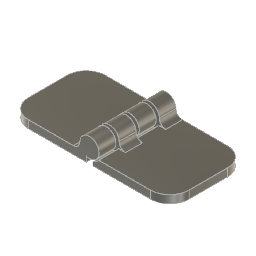
hinge (Autodesk Fusion 360 design; units mm, degrees)
Autodesk Fusion 360 part; units mm, degrees
note: some values were not read from the file. Set by a fixed rule: which sketch regions a step uses.
sketch "Sketch1" plane through (0, 0, 0) normal (0, 0, 1) x (1, 0, 0)
  line L0 (25, -12) -> (-25, -12) construction
  line L1 (-25, -6) -> (-25, 6) construction
  line L2 (-25, 12) -> (25, 12) construction
  line L3 (25, 6) -> (25, -12) construction
  line L4 (25, -12) -> (-25, 12) construction
  line L5 (-25, -12) -> (25, 12) construction
  line L6 (0, 12) -> (0, -12) construction
  line L7 (-19, 12) -> (-1, 12)
  line L8 (-1, 12) -> (-1, -12)
  line L9 (-1, -12) -> (-19, -12)
  line L10 (-25, -12) -> (-25, 12)
  line L11 (1, 12) -> (19, 12)
  line L12 (25, 12) -> (25, -6)
  line L13 (19, -12) -> (1, -12)
  line L14 (1, -12) -> (1, 12)
  arc A0 (-19, 12) -> (-25, 6) centre (-19, 6) ccw
  arc A1 (-25, -6) -> (-19, -12) centre (-19, -6) ccw
  arc A2 (19, -12) -> (25, -6) centre (19, -6) ccw
  arc A3 (25, 6) -> (19, 12) centre (19, 6) ccw
  dimension "d1" = 6
  dimension "d2" = 6
  dimension "d3" = 6
  constraint horizontal L0
  constraint perpendicular L0 L1
  constraint parallel L0 L2
  constraint parallel L1 L3
  constraint coincident L4 origin
  constraint coincident L5 origin
  constraint midpoint L2 L6.start
  constraint midpoint L0 L6.end
  constraint horizontal L7
  constraint vertical L8
  constraint horizontal L9
  constraint vertical L10
  constraint coincident L0 L8.end
  constraint horizontal L11
  constraint vertical L12
  constraint horizontal L13
  constraint vertical L14
  constraint coincident L2.start L1
  constraint coincident L2.start L7
  constraint tangent L1 A0
  constraint tangent L7 A0
  constraint coincident L0.end L1
  constraint coincident L0.end L9
  constraint tangent L1 A1
  constraint tangent L9 A1
  constraint coincident L0.start L13
  constraint coincident L0.start L12
  constraint tangent L13 A2
  constraint tangent L12 A2
  constraint coincident L2.end L11
  constraint coincident L2.end L3
  constraint tangent L11 A3
  constraint tangent L3 A3
  constraint equal A2 A3
  measures "d1" radius of A0
  measures "d2" radius of A1
  measures "d3" radius of A2
extrude "Extrude1" add sketch "Sketch1" along normal blind 2.5 makes body 1 at (-7, -4, 0) makes body 2 at (7, 4, 0)
sketch "Sketch2" plane through (0, 12, 0) normal (0, 1, 0) x (1, 0, 0)
  line L0 (-19, -2.5) -> (-5, -2.5)
  circle A0 centre (0, -4.5) radius 3
  circle A1 centre (0, -4.5) radius 1.5
  line L1 (-3, -4.5) -> (-3, -4.5) construction
  line L2 (3, -4.5) -> (3, -4.5) construction
  arc A2 (-3, -4.5) -> (-5, -2.5) centre (-5, -4.5) ccw
  line L3 (5, -2.5) -> (7.5, -2.5) construction
  arc A3 (5, -2.5) -> (3, -4.5) centre (5, -4.5) ccw
  line L4 (-5, -2.5) -> (5, -2.5)
  circle A4 centre (0, -4.5) radius 1.25
  line L5 (-1, 0) -> (-19, 0)
  line L6 (-19, 0) -> (-19, -2.5)
  line L7 (-19, -2.5) -> (-1, -2.5)
  line L8 (-1, -2.5) -> (-1, 0)
  point P0 (19, -2.5)
  dimension "d6" = 38
  dimension "d7" = 6
  dimension "d8" = 3
  dimension "d9" = 2
  dimension "d10" = 2
  dimension "d11" = 2.5
  constraint horizontal L0
  constraint concentric A0 A1
  constraint coincident A0 L1.start
  constraint coincident A0 L2.start
  constraint coincident P0 L0
  constraint tangent L0 A2
  constraint tangent A2 L3
  constraint coincident L0.end L3
  constraint tangent L3 A3
  constraint concentric A0 A4
  measures "d6" distance of L0.start P0
  measures "d7" diameter of A0
  measures "d8" diameter of A1
  measures "d9" radius of A2
  measures "d10" radius of A3
  measures "d11" diameter of A4
extrude "Extrude2" add sketch "Sketch2" against normal blind 5.25 contours A0 A2 L4 L7 | A0 L4 L7 | A0 A3 L4 bodies 1 2
extrude "Extrude3" add sketch "Sketch2" against normal blind 5.25 from surface at -6.25 contours A0 A2 L4 L7 | A0 L4 L7 | A0 A3 L4 | A1 bodies 1
extrude "Extrude4" add sketch "Sketch2" against normal blind 5.25 from surface at -12.5 contours A0 A2 L4 L7 | A0 L4 L7 | A0 A3 L4 bodies 1
extrude "Extrude5" add sketch "Sketch2" against normal blind 5.25 from surface at -18.75 contours A0 A2 L4 L7 | A0 L4 L7 | A0 A3 L4 | A1 bodies 1
extrude "Extrude6" add sketch "Sketch2" against normal blind 24 contours A4 bodies 1
sketch "Sketch3" plane through (0, 12, 5.583) normal (0, 1, 0) x (1, 0, 0)
sketch "Sketch4" plane through (0, 12, 0) normal (0, 1, 0) x (1, 0, 0)
  circle A0 centre (0, -4.5) radius 1
  dimension "d25" = 2
  measures "d25" diameter of A0
extrude "Extrude7" cut sketch "Sketch2" against normal blind 24 contours A4 bodies 1
extrude "Extrude8" add sketch "Sketch2" against normal blind 5.25 from surface at -6.25 contours A4 bodies 1
extrude "Extrude9" add sketch "Sketch2" against normal blind 5.25 from surface at -18.75 contours A4 bodies 1
extrude "Extrude10" add sketch "Sketch4" against normal blind 24 bodies 1
extrude "Extrude11" cut sketch "Sketch2" against normal blind 5.25 contours A0 A2 L4 L7 bodies 1
extrude "Extrude12" cut sketch "Sketch2" against normal blind 5.25 from surface at -12.5 contours A0 A2 L4 L7 bodies 1
extrude "Extrude13" cut sketch "Sketch2" against normal blind 5.25 from surface at -6.25 contours A0 A3 L4 bodies 1
extrude "Extrude14" cut sketch "Sketch2" against normal blind 5.25 from surface at -18.75 contours A0 A3 L4 bodies 1
extrude "Extrude15" add sketch "Sketch2" against normal blind 5.25 contours A0 L4 L7 L8 | A0 L4 L8 bodies 1
extrude "Extrude16" add sketch "Sketch2" against normal blind 5.25 from surface at -6.25 contours A0 L4 L7 L8 | A0 L4 L8 bodies 1
extrude "Extrude17" add sketch "Sketch2" against normal blind 5.25 from surface at -12.5 contours A0 L4 L7 L8 | A0 L4 L8 bodies 1
extrude "Extrude18" add sketch "Sketch2" against normal blind 5.25 from surface at -18.75 contours A0 L4 L7 L8 | A0 L4 L8 bodies 1
sketch "Sketch5" plane through (0, 12, 0) normal (0, 1, 0) x (1, 0, 0)
  circle A0 centre (0, -4.5) radius 3
  circle A1 centre (0, -4.5) radius 3.5
  line L0 (-1, -2.5) -> (-3.5, -2.5)
  line L1 (-3.5, -2.5) -> (-3.5, -0.7)
  line L2 (-3.5, -0.7) -> (-1, -0.7)
  line L3 (-1, -0.7) -> (-1, -2.5)
  line L4 (1, -0.7) -> (3.5, -0.7)
  line L5 (3.5, -0.7) -> (3.5, -2.5)
  line L6 (3.5, -2.5) -> (1, -2.5)
  line L7 (1, -2.5) -> (1, -0.7)
  dimension "d58" = 6
  dimension "d59" = 7
  constraint concentric A0 A1
  constraint horizontal L0
  constraint vertical L1
  constraint horizontal L2
  constraint vertical L3
  constraint horizontal L4
  constraint vertical L5
  constraint horizontal L6
  constraint vertical L7
  measures "d58" diameter of A0
  measures "d59" diameter of A1
extrude "Extrude19" cut sketch "Sketch5" against normal blind 6.25 contours A0 A1 L0 L3 bodies 1
extrude "Extrude20" cut sketch "Sketch5" against normal blind 7.25 from surface at -11.5 contours A0 A1 L0 L3 bodies 1
extrude "Extrude21" cut sketch "Sketch5" against normal blind 1 from surface at -5.25 contours A0 L6 L7 | A0 L0 L3 bodies 1
extrude "Extrude22" cut sketch "Sketch5" against normal blind 1 from surface at -11.5 contours A0 L6 L7 | A0 L0 L3 bodies 1
extrude "Extrude23" cut sketch "Sketch5" against normal blind 1 from surface at -17.75 contours A0 L6 L7 | A0 L0 L3 bodies 1
extrude "Extrude24" cut sketch "Sketch5" against normal blind 7.25 from surface at -5.25 contours A0 A1 L6 L7 bodies 1
extrude "Extrude25" cut sketch "Sketch5" against normal blind 6.25 from surface at -17.75 contours A0 A1 L6 L7 bodies 1 makes body 3 at (7, 4, 0)
